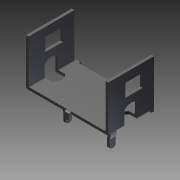
# Autodesk Inventor part: AS11CHra1
Saved by Autodesk Inventor 2011 SP1 (Build 150282100, 282)
## iProperties
Created: 2018-06-01
Part Number: AS11CHra1
Catalog Web Link: www.cadenas.de
Description: AS - Series - Bracket for Right Angle - Poles 1 & 2-
Vendor: NKKSWITCHES
Document SubType Name: Modeling
Designer: psAdmin
Manufacturer: NKKSWITCHES
Mass: 0.0294174 g
Surface Area: 2.2239 cm^2
Volume: 0.0294174 cm^3
Density: 1 g/cm^3
Category: PARTsolutions
Company: NKKSWITCHES
Title: AS11CHra1
Author: Cadenas PARTsolutions
PSOL_IDENT_0: {$CADENAS_DATA\23d-libs\nkkswitches\slides\as\parts\as_bracket_ra1.prj},226 {VTYP=3D},{NB=AS11CHra1}
PSOL_IDENT_1: ,{LINA=AS11CHra1},{NN=AS - Series - Bracket for Right Angle - Poles 1 & 2},{DATE=11.10.2017 10:53:50
PSOL_IDENT_2: },{GEOMDATE=09.12.2008 09:50:00},{VERSION=},{LINEID=10},{LINESUBID=-1},{WBVAR=PLS,CRCTS,ACTU,TRMNLS}
PSOL_IDENT_3: {NB=AS11CHra1},{LINA=AS11CHra1},{KT=DUMMY},{PN=AS11CH},{SRS=AS},{PLS=1},{CRCTS=1},{ACTU=C},{TRMNLS=
PSOL_IDENT_4: H},{CRCTSALG=  '1', '1 - ON/NONE/OFF','2', '2 - ON/NONE/ON', '3', '3 - ON/OFF/ON' }
NN: AS - Series - Bracket for Right Angle - Poles 1 & 2
NB: AS11CHra1
NBSYN: $PN.ra1
LINA: AS11CHra1
PN: AS11CH
SRS: AS
PLS: 1 - SPST/SPDT
CRCTS: 1 - ON/NONE/OFF
ACTU: C - .150"(3,8mm)Long
TRMNLS: H - Right Angle with Bracket
SUPPLIER: NKKSWITCHES
ARTICLENO: AS11CHra1
BOMINFO: AS11CHra1
CREATOR: CADENAS GmbH
Autodesk Inventor part; units mm, degrees
sketch "Sketch_1" plane through (0, 0, 0) normal (0, 0, 1) x (1, 0, 0)
  arc A0 (0, 0.1524) -> (0.1524, 0) centre (0.1524, 0.1524) ccw
  line L0 (0.1524, 0) -> (9.4488, 0)
  arc A1 (9.4488, 0) -> (9.6012, 0.1524) centre (9.4488, 0.1524) ccw
  line L1 (9.6012, 0.1524) -> (9.6012, 5.3848)
  line L2 (9.6012, 5.3848) -> (9.2964, 5.3848)
  line L3 (9.2964, 5.3848) -> (9.2964, 0.4572)
  arc A2 (9.144, 0.3048) -> (9.2964, 0.4572) centre (9.144, 0.4572) ccw
  line L4 (9.144, 0.3048) -> (0.4572, 0.3048)
  arc A3 (0.3048, 0.4572) -> (0.4572, 0.3048) centre (0.4572, 0.4572) ccw
  line L5 (0.3048, 0.4572) -> (0.3048, 5.3848)
  line L6 (0.3048, 5.3848) -> (0, 5.3848)
  line L7 (0, 5.3848) -> (0, 0.1524)
  constraints: 16 end point, 8 point on circle, 4 centre point
extrude "Extrusion1" add sketch "Sketch_1" along normal blind 5.334
sketch "Sketch_3" plane through (0, 0, 2.3622) normal (0, 0, 1) x (1, 0, 0)
  arc A0 (2.1031, -1.0313) -> (2.1031, -2.5501) centre (4.4075, -1.7907) ccw
  arc A1 (2.1082, -2.5819) -> (2.1031, -2.5501) centre (2.0066, -2.5819) ccw
  line L0 (2.1082, -2.5819) -> (2.1082, -3.5814)
  line L1 (2.1082, -3.5814) -> (2.413, -3.5814)
  line L2 (2.413, -3.5814) -> (2.413, -2.5819)
  arc A2 (2.413, -2.5819) -> (2.4079, -2.5501) centre (2.3114, -2.5819) ccw
  arc A3 (2.4079, -1.0313) -> (2.4079, -2.5501) centre (4.7123, -1.7907) ccw
  arc A4 (2.4079, -1.0313) -> (2.413, -0.9995) centre (2.3114, -0.9995) ccw
  line L3 (2.413, -0.9995) -> (2.413, 0)
  line L4 (2.413, 0) -> (2.1082, 0)
  line L5 (2.1082, 0) -> (2.1082, -0.9995)
  arc A5 (2.1031, -1.0313) -> (2.1082, -0.9995) centre (2.0066, -0.9995) ccw
  constraints: 12 end point, 12 point on circle, 6 centre point
extrude "Extrusion2" add sketch "Sketch_3" along normal blind 0.7112
sketch "Sketch_4" plane through (0, 0, 2.3622) normal (0, 0, 1) x (1, 0, 0)
  arc A0 (7.1882, -0.9995) -> (7.1933, -1.0313) centre (7.2898, -0.9995) ccw
  arc A1 (7.1933, -2.5501) -> (7.1933, -1.0313) centre (4.8889, -1.7907) ccw
  arc A2 (7.1933, -2.5501) -> (7.1882, -2.5819) centre (7.2898, -2.5819) ccw
  line L0 (7.1882, -2.5819) -> (7.1882, -3.5814)
  line L1 (7.1882, -3.5814) -> (7.493, -3.5814)
  line L2 (7.493, -3.5814) -> (7.493, -2.5819)
  arc A3 (7.4981, -2.5501) -> (7.493, -2.5819) centre (7.5946, -2.5819) ccw
  arc A4 (7.4981, -2.5501) -> (7.4981, -1.0313) centre (5.1937, -1.7907) ccw
  arc A5 (7.493, -0.9995) -> (7.4981, -1.0313) centre (7.5946, -0.9995) ccw
  line L3 (7.493, -0.9995) -> (7.493, 0)
  line L4 (7.493, 0) -> (7.1882, 0)
  line L5 (7.1882, 0) -> (7.1882, -0.9995)
  constraints: 12 end point, 12 point on circle, 6 centre point
extrude "Extrusion3" add sketch "Sketch_4" along normal blind 0.7112
sketch "Sketch_5" plane through (0, 0, 0) normal (1, 0, 0) x (0, 1, 0)
  line L0 (-3.3274, 3.0734) -> (-3.8354, 3.0734)
  line L1 (-3.8354, 3.0734) -> (-3.8354, 2.3622)
  line L2 (-3.8354, 2.3622) -> (-3.3274, 2.3622)
  arc A0 (-3.3274, 3.0734) -> (-3.3274, 2.3622) centre (-3.2408, 2.7178) ccw
  constraints: 6 end point, 2 point on circle, 1 centre point
extrude "Extrusion4" cut sketch "Sketch_5" along normal blind 8.3058
sketch "Sketch_6" plane through (0, 0, 0) normal (1, 0, 0) x (0, 1, 0)
  line L0 (2.8448, 3.3655) -> (2.8448, 1.3335)
  line L1 (2.8448, 1.3335) -> (4.3688, 1.3335)
  line L2 (4.3688, 1.3335) -> (4.3688, 3.3655)
  line L3 (4.3688, 3.3655) -> (2.8448, 3.3655)
  constraints: 8 end point
extrude "Extrusion5" cut sketch "Sketch_6" along normal blind 10.16
sketch "Sketch_7" plane through (0, 0, 0) normal (1, 0, 0) x (0, 1, 0)
  line L0 (1.651, 3.4449) -> (0, 3.4449)
  line L1 (0, 3.4449) -> (0, 1.9209)
  line L2 (0, 1.9209) -> (1.651, 1.9209)
  arc A0 (1.651, 1.9209) -> (1.651, 3.4449) centre (1.0795, 2.6829) ccw
  constraints: 6 end point, 2 point on circle, 1 centre point
extrude "Extrusion6" cut sketch "Sketch_7" along normal blind 0.3048
sketch "Sketch_8" plane through (9.8044, 0, 0) normal (1, 0, 0) x (0, 0, -1)
  line L0 (-3.4449, 1.651) -> (-3.4449, 0)
  line L1 (-3.4449, 0) -> (-1.9209, 0)
  line L2 (-1.9209, 0) -> (-1.9209, 1.651)
  arc A0 (-1.9209, 1.651) -> (-3.4449, 1.651) centre (-2.6829, 1.0795) ccw
  constraints: 6 end point, 2 point on circle, 1 centre point
extrude "Extrusion7" cut sketch "Sketch_8" against normal blind 0.508
sketch "Sketch_9" plane through (0, 0, 0) normal (0, 1, 0) x (-1, 0, 0)
  line L0 (0, 1.9209) -> (0, 3.4449)
  line L1 (0, 3.4449) -> (-1.143, 3.4449)
  arc A0 (-1.143, 3.4449) -> (-1.143, 1.9209) centre (-0.5715, 2.6829) ccw
  line L2 (-1.143, 1.9209) -> (0, 1.9209)
  constraints: 6 end point, 2 point on circle, 1 centre point
extrude "Extrusion8" cut sketch "Sketch_9" along normal blind 0.508
sketch "Sketch_10" plane through (0, 0, 0) normal (0, 1, 0) x (-1, 0, 0)
  arc A0 (-8.6614, 1.9209) -> (-8.6614, 3.4449) centre (-9.2329, 2.6829) ccw
  line L0 (-8.6614, 3.4449) -> (-9.8044, 3.4449)
  line L1 (-9.8044, 3.4449) -> (-9.8044, 1.9209)
  line L2 (-9.8044, 1.9209) -> (-8.6614, 1.9209)
  constraints: 6 end point, 2 point on circle, 1 centre point
extrude "Extrusion9" cut sketch "Sketch_10" along normal blind 0.508
sketch "Sketch_11" plane through (0.3048, 0, 0) normal (1, 0, 0) x (0, 0, -1)
  line L0 (0, -0.4826) -> (0.3048, -0.4826)
  line L1 (0.3048, -0.4826) -> (0.3048, 0.1778)
  arc A0 (0.3048, 0.1778) -> (0.1778, 0.3048) centre (0.1778, 0.1778) ccw
  line L2 (0.1778, 0.3048) -> (0, 0.3048)
  line L3 (0, 0.3048) -> (0, -0.4826)
  constraints: 8 end point, 2 point on circle, 1 centre point
extrude "Extrusion10" add sketch "Sketch_11" along normal blind 0.508
sketch "Sketch_12" plane through (9.2964, 0, 0) normal (1, 0, 0) x (0, 0, -1)
  line L0 (0, -0.4826) -> (0.3048, -0.4826)
  line L1 (0.3048, -0.4826) -> (0.3048, 0.1778)
  arc A0 (0.3048, 0.1778) -> (0.1778, 0.3048) centre (0.1778, 0.1778) ccw
  line L2 (0.1778, 0.3048) -> (0, 0.3048)
  line L3 (0, 0.3048) -> (0, -0.4826)
  constraints: 8 end point, 2 point on circle, 1 centre point
extrude "Extrusion11" add sketch "Sketch_12" against normal blind 0.508
sketch "Sketch_13" plane through (4.8006, 0, 0) normal (1, 0, 0) x (0, 0, -1)
  line L0 (-5.6388, -0.4826) -> (-5.334, -0.4826)
  line L1 (-5.334, -0.4826) -> (-5.334, 0.3048)
  line L2 (-5.334, 0.3048) -> (-5.5118, 0.3048)
  arc A0 (-5.5118, 0.3048) -> (-5.6388, 0.1778) centre (-5.5118, 0.1778) ccw
  line L3 (-5.6388, 0.1778) -> (-5.6388, -0.4826)
  constraints: 8 end point, 2 point on circle, 1 centre point
extrude "Extrusion12" add sketch "Sketch_13" along normal blind 0.508
ref_plane "cp_right_body_pole1_XY" through (4.8006, 0.3048, 3.3655) normal (0, -1, 0) x (1, 0, 0)
ref_plane "cp_right_body_pole1_YZ" through (4.8006, 0.3048, 3.3655) normal (1, 0, 0) x (0, 0, 1)
ref_plane "cp_right_body_pole1_ZX" through (4.8006, 0.3048, 3.3655) normal (0, 0, 1) x (0, -1, 0)
body "Solid1"
